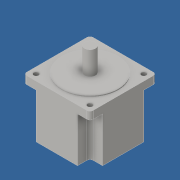
# Autodesk Inventor part: Nema34
Saved by Autodesk Inventor 2016 (Build 200138000, 138)
## iProperties
Created: 2015-08-24
Part Number: Nema34
Material: Generisch
Document SubType Name: Modeling
Designer: 4ndreas
Density: 1 g/cm^3
Appearance: Vorgabe
Author: 4ndreas
Autodesk Inventor part; units mm, degrees
ref_plane "YZ Plane" through (0, 0, 0) normal (1, 0, 0) x (0, 1, 0)
ref_plane "XZ Plane" through (0, 0, 0) normal (0, 1, 0) x (-1, 0, 0)
ref_plane "XY Plane" through (0, 0, 0) normal (0, 0, 1) x (1, 0, 0)
sketch "Skizze1" plane through (0, 0, 0) normal (0, 0, 1) x (1, 0, 0)
  line L0 (-38.9, -42.9) -> (38.9, -42.9)
  line L1 (42.9, -38.9) -> (42.9, 38.9)
  line L2 (38.9, 42.9) -> (-38.9, 42.9)
  line L3 (-42.9, 38.9) -> (-42.9, -38.9)
  line L4 (-42.9, -42.9) -> (42.9, 42.9) construction
  line L5 (42.9, -42.9) -> (-42.9, 42.9) construction
  arc A0 (42.9, 38.9) -> (38.9, 42.9) centre (38.9, 38.9) ccw
  arc A1 (38.9, -42.9) -> (42.9, -38.9) centre (38.9, -38.9) ccw
  arc A2 (-42.9, -38.9) -> (-38.9, -42.9) centre (-38.9, -38.9) ccw
  arc A3 (-38.9, 42.9) -> (-42.9, 38.9) centre (-38.9, 38.9) ccw
  point P0 (0, 0)
  dimension "d0" = 4
  dimension "d1" = 85.8
  constraints: 12 end point, 8 point on circle, 8 point on line, 8 tangent, 4 centre point, 3 equal radius, 2 midpoint, 2 parallel, 2 perpendicular, 1 horizontal
  measures "d0" radius of A0
  measures "d1" distance between parallel lines of L0 L2
extrude "Extrusion1" add sketch "Skizze1" against normal blind 10
sketch "Skizze2" plane through (0, 0, 0) normal (0, 0, 1) x (1, 0, 0)
  circle A0 centre (0, 0) radius 36.5
  dimension "d4" = 73
  constraints: 1 centre point, 1 coincident
  measures "d4" diameter of A0
extrude "Extrusion2" add sketch "Skizze2" along normal blind 1.6
sketch "Skizze3" plane through (0, 0, -10) normal (0, 0, -1) x (-1, 0, 0)
  line L0 (-42.9, 38.9) -> (-42.9, -38.9) projected
  arc A0 (-42.9, -38.9) -> (-38.9, -42.9) centre (-38.9, -38.9) ccw projected
  line L1 (-38.9, -42.9) -> (38.9, -42.9) projected
  arc A1 (38.9, -42.9) -> (42.9, -38.9) centre (38.9, -38.9) ccw projected
  line L2 (42.9, -38.9) -> (42.9, 38.9) projected
  arc A2 (42.9, 38.9) -> (38.9, 42.9) centre (38.9, 38.9) ccw projected
  line L3 (38.9, 42.9) -> (-38.9, 42.9) projected
  arc A3 (-38.9, 42.9) -> (-42.9, 38.9) centre (-38.9, 38.9) ccw projected
  line L4 (42.9, -26.7) -> (30.7, -26.7)
  line L5 (26.7, -30.7) -> (26.7, -42.9)
  arc A4 (30.7, -26.7) -> (26.7, -30.7) centre (30.7, -30.7) ccw
  line L6 (38.9, -38.9) -> (-38.9, 38.9) construction
  circle A5 centre (34.8, -34.8) radius 8.1 construction
  line L7 (38.9, 38.9) -> (-38.9, -38.9) construction
  line L8 (34.8, -34.8) -> (-34.8, -34.8) construction
  line L9 (42.9, -38.9) -> (42.9, 38.9) projected
  line L10 (42.9, -26.7) -> (42.9, -38.9)
  line L11 (-38.9, -42.9) -> (38.9, -42.9) projected
  line L12 (26.7, -42.9) -> (38.9, -42.9)
  arc A6 (38.9, -42.9) -> (42.9, -38.9) centre (38.9, -38.9) ccw
  arc A7 (42.9, 38.9) -> (38.9, 42.9) centre (38.9, 38.9) ccw
  line L13 (42.9, 26.7) -> (42.9, 38.9)
  line L14 (30.7, 26.7) -> (42.9, 26.7)
  arc A8 (26.7, 30.7) -> (30.7, 26.7) centre (30.7, 30.7) ccw
  line L15 (26.7, 42.9) -> (26.7, 30.7)
  line L16 (26.7, 42.9) -> (38.9, 42.9)
  arc A9 (-38.9, 42.9) -> (-42.9, 38.9) centre (-38.9, 38.9) ccw
  line L17 (-26.7, 42.9) -> (-38.9, 42.9)
  line L18 (-26.7, 30.7) -> (-26.7, 42.9)
  arc A10 (-30.7, 26.7) -> (-26.7, 30.7) centre (-30.7, 30.7) ccw
  line L19 (-42.9, 26.7) -> (-30.7, 26.7)
  line L20 (-42.9, 26.7) -> (-42.9, 38.9)
  arc A11 (-42.9, -38.9) -> (-38.9, -42.9) centre (-38.9, -38.9) ccw
  line L21 (-42.9, -26.7) -> (-42.9, -38.9)
  line L22 (-30.7, -26.7) -> (-42.9, -26.7)
  arc A12 (-26.7, -30.7) -> (-30.7, -26.7) centre (-30.7, -30.7) ccw
  line L23 (-26.7, -42.9) -> (-26.7, -30.7)
  line L24 (-26.7, -42.9) -> (-38.9, -42.9)
  point P0 (0, 0)
  dimension "d7" = 4
  dimension "d8" = 69.6
  dimension "d11" = 360
  constraints: 38 end point, 16 point on circle, 9 centre point, 6 tangent, 5 point on line, 2 collinear, 2 horizontal, 1 perpendicular, 57 other
  measures "d7" radius of A4
  measures "d8" distance of L8.start L8.end
extrude "Extrusion3" add sketch "Skizze3" along normal blind 58 contours L19 A10 L18 L3 L15 A8 L14 L2 L4 A4 L5 L1 L23 A12 L22 L0
sketch "Skizze4" plane through (0, 0, 0) normal (0, 0, 1) x (1, 0, 0)
  circle A0 centre (0, 0) radius 36.5 projected
  line L0 (42.9, 38.9) -> (42.9, -38.9) projected
  arc A1 (42.9, 38.9) -> (38.9, 42.9) centre (38.9, 38.9) ccw projected
  line L1 (-38.9, 42.9) -> (38.9, 42.9) projected
  arc A2 (-38.9, 42.9) -> (-42.9, 38.9) centre (-38.9, 38.9) ccw projected
  line L2 (-42.9, -38.9) -> (-42.9, 38.9) projected
  arc A3 (-42.9, -38.9) -> (-38.9, -42.9) centre (-38.9, -38.9) ccw projected
  line L3 (38.9, -42.9) -> (-38.9, -42.9) projected
  arc A4 (38.9, -42.9) -> (42.9, -38.9) centre (38.9, -38.9) ccw projected
  line L4 (38.9, -38.9) -> (-38.9, 38.9) construction
  line L5 (-34.8, 34.8) -> (34.8, 34.8) construction
  line L6 (34.8, 34.8) -> (34.8, -34.8) construction
  line L7 (34.8, -34.8) -> (-34.8, -34.8) construction
  line L8 (-34.8, -34.8) -> (-34.8, 34.8) construction
  line L9 (-34.8, 34.8) -> (34.8, -34.8) construction
  line L10 (34.8, 34.8) -> (-34.8, -34.8) construction
  dimension "d15" = 69.6
  constraints: 14 end point, 2 midpoint, 2 parallel, 1 horizontal, 1 perpendicular, 1 point on line
  measures "d15" distance between parallel lines of L8 L6
hole "Bohrung1" at (34.8, 34.8, 0) at (-34.8, 34.8, 0) at (-34.8, -34.8, 0) at (34.8, -34.8, 0) direction (0, 0, -1) diameter 6.5 end through all
sketch "Skizze5" plane through (0, 0, 1.6) normal (0, 0, 1) x (1, 0, 0)
  circle A0 centre (0, 0) radius 7
  dimension "d23" = 14
  constraints: 1 centre point, 1 coincident
  measures "d23" diameter of A0
extrude "Extrusion4" add sketch "Skizze5" along normal blind 30.4
